Autodesk Fusion 360 part; units mm, degrees
(part 6 of 8)
  spline S293 degree 5 poles (-65.7422, 42.7079) (-65.7471, 42.7094) (-65.7716, 42.7166) (-65.8155, 42.7296) (-65.8791, 42.7481) (-65.9624, 42.7721) (-66.0605, 42.7999) (-66.1588, 42.8273) (-66.2573, 42.8543) (-66.356, 42.8809) (-66.4549, 42.9071) (-66.5539, 42.9329) (-66.6532, 42.9583) (-66.7526, 42.9833) (-66.8522, 43.008) (-66.9519, 43.0322) (-67.0519, 43.0561) (-67.152, 43.0797) (-67.2522, 43.1028) (-67.3527, 43.1256) (-67.4532, 43.148) (-67.554, 43.1701) (-67.6549, 43.1918) (-67.756, 43.2132) (-67.8572, 43.2342) (-67.9585, 43.2548) (-68.06, 43.2752) (-68.1617, 43.2951) (-68.2635, 43.3147) (-68.3654, 43.334) (-68.4675, 43.353) (-68.5697, 43.3716) (-68.6721, 43.3898) (-68.7746, 43.4078) (-68.8772, 43.4254) (-68.98, 43.4426) (-69.0829, 43.4596) (-69.1859, 43.4762) (-69.289, 43.4925) (-69.3716, 43.5053) (-69.4337, 43.5147) (-69.475, 43.521) (-69.4957, 43.524) knots 0.467834 0.467834 0.467834 0.467834 0.467834 0.467834 0.471429 0.485714 0.5 0.514286 0.528571 0.542857 0.557143 0.571429 0.585714 0.6 0.614286 0.628571 0.642857 0.657143 0.671429 0.685714 0.7 0.714286 0.728571 0.742857 0.757143 0.771429 0.785714 0.8 0.814286 0.828571 0.842857 0.857143 0.871429 0.885714 0.9 0.914286 0.928571 0.942857 0.957143 0.971429 0.985714 1 1 1 1 1 1
  arc A147 (-69.4957, 43.524) -> (-70.3306, 42.1616) centre (0, 0) ccw
  spline S294 degree 5 poles (-70.3306, 42.1616) (-70.3185, 42.1446) (-70.2941, 42.1106) (-70.2576, 42.0596) (-70.2087, 41.9918) (-70.1473, 41.9073) (-70.0857, 41.823) (-70.0239, 41.7391) (-69.9619, 41.6553) (-69.8996, 41.5719) (-69.8371, 41.4887) (-69.7743, 41.4058) (-69.7114, 41.3232) (-69.6481, 41.2408) (-69.5847, 41.1587) (-69.521, 41.0769) (-69.457, 40.9954) (-69.3929, 40.9142) (-69.3285, 40.8333) (-69.2638, 40.7526) (-69.1989, 40.6723) (-69.1337, 40.5922) (-69.0683, 40.5125) (-69.0027, 40.433) (-68.9368, 40.3539) (-68.8706, 40.2751) (-68.8042, 40.1966) (-68.7376, 40.1184) (-68.6706, 40.0405) (-68.6035, 39.963) (-68.536, 39.8857) (-68.4683, 39.8088) (-68.4004, 39.7323) (-68.3321, 39.6561) (-68.2636, 39.5802) (-68.1949, 39.5047) (-68.1258, 39.4296) (-68.0565, 39.3548) (-67.9974, 39.2915) (-67.9519, 39.2433) (-67.9204, 39.21) (-67.9029, 39.1915) (-67.8994, 39.1878) knots -1 -1 -1 -1 -1 -1 -0.985714 -0.971429 -0.957143 -0.942857 -0.928571 -0.914286 -0.9 -0.885714 -0.871429 -0.857143 -0.842857 -0.828571 -0.814286 -0.8 -0.785714 -0.771429 -0.757143 -0.742857 -0.728571 -0.714286 -0.7 -0.685714 -0.671429 -0.657143 -0.642857 -0.628571 -0.614286 -0.6 -0.585714 -0.571429 -0.557143 -0.542857 -0.528571 -0.514286 -0.5 -0.485714 -0.471429 -0.467834 -0.467834 -0.467834 -0.467834 -0.467834 -0.467834
  spline S295 degree 3 poles (-67.7523, 38.0098) (-67.6886, 38.1234) (-67.6476, 38.2483) (-67.616, 38.5068) (-67.6256, 38.6379) (-67.6817, 38.8427) (-67.7131, 38.9189) (-67.7938, 39.0619) (-67.8428, 39.1282) (-67.8994, 39.1878) knots 0 0 0 0 0.039064 0.039064 0.078129 0.078129 0.102767 0.102767 0.127404 0.127404 0.127404 0.127404
  arc A148 (-67.7523, 38.0098) -> (-67.8091, 37.9083) centre (0, 0) ccw
  spline S296 degree 3 poles (-68.8904, 37.4182) (-68.763, 37.391) (-68.6316, 37.389) (-68.3754, 37.4355) (-68.253, 37.4836) (-68.0741, 37.598) (-68.0106, 37.6506) (-67.898, 37.7701) (-67.8492, 37.8366) (-67.8091, 37.9083) knots 0 0 0 0 0.039064 0.039064 0.078129 0.078129 0.102767 0.102767 0.127404 0.127404 0.127404 0.127404
  spline S297 degree 5 poles (-68.8904, 37.4182) (-68.8954, 37.4192) (-68.9203, 37.4245) (-68.9652, 37.434) (-69.03, 37.4475) (-69.1149, 37.4649) (-69.2149, 37.4849) (-69.315, 37.5045) (-69.4153, 37.5237) (-69.5158, 37.5425) (-69.6164, 37.5608) (-69.7172, 37.5788) (-69.8182, 37.5963) (-69.9192, 37.6135) (-70.0204, 37.6302) (-70.1218, 37.6466) (-70.2233, 37.6626) (-70.3249, 37.6782) (-70.4267, 37.6934) (-70.5286, 37.7082) (-70.6307, 37.7227) (-70.7328, 37.7368) (-70.8351, 37.7505) (-70.9376, 37.7639) (-71.0401, 37.7769) (-71.1428, 37.7895) (-71.2456, 37.8018) (-71.3485, 37.8137) (-71.4515, 37.8253) (-71.5546, 37.8365) (-71.6579, 37.8474) (-71.7612, 37.8579) (-71.8647, 37.8681) (-71.9683, 37.878) (-72.072, 37.8875) (-72.1758, 37.8966) (-72.2797, 37.9054) (-72.3837, 37.9139) (-72.4878, 37.9221) (-72.5712, 37.9283) (-72.6338, 37.9329) (-72.6755, 37.9358) (-72.6964, 37.9373) knots 0.467834 0.467834 0.467834 0.467834 0.467834 0.467834 0.471429 0.485714 0.5 0.514286 0.528571 0.542857 0.557143 0.571429 0.585714 0.6 0.614286 0.628571 0.642857 0.657143 0.671429 0.685714 0.7 0.714286 0.728571 0.742857 0.757143 0.771429 0.785714 0.8 0.814286 0.828571 0.842857 0.857143 0.871429 0.885714 0.9 0.914286 0.928571 0.942857 0.957143 0.971429 0.985714 1 1 1 1 1 1
  arc A149 (-72.6964, 37.9373) -> (-73.4218, 36.5136) centre (0, 0) ccw
  spline S298 degree 5 poles (-73.4218, 36.5136) (-73.4083, 36.4976) (-73.3814, 36.4656) (-73.3409, 36.4176) (-73.2869, 36.3538) (-73.2191, 36.2744) (-73.1511, 36.1952) (-73.0829, 36.1164) (-73.0144, 36.0378) (-72.9458, 35.9595) (-72.877, 35.8815) (-72.8079, 35.8037) (-72.7386, 35.7263) (-72.6692, 35.6491) (-72.5995, 35.5723) (-72.5295, 35.4958) (-72.4594, 35.4195) (-72.389, 35.3436) (-72.3185, 35.2679) (-72.2477, 35.1926) (-72.1767, 35.1176) (-72.1054, 35.0429) (-72.034, 34.9686) (-71.9623, 34.8945) (-71.8904, 34.8208) (-71.8183, 34.7474) (-71.7459, 34.6743) (-71.6733, 34.6016) (-71.6005, 34.5292) (-71.5274, 34.4572) (-71.4541, 34.3855) (-71.3806, 34.3142) (-71.3069, 34.2432) (-71.2329, 34.1726) (-71.1586, 34.1023) (-71.0842, 34.0324) (-71.0094, 33.9629) (-70.9345, 33.8938) (-70.8705, 33.8353) (-70.8215, 33.7908) (-70.7874, 33.7601) (-70.7685, 33.7431) (-70.7647, 33.7396) knots -1 -1 -1 -1 -1 -1 -0.985714 -0.971429 -0.957143 -0.942857 -0.928571 -0.914286 -0.9 -0.885714 -0.871429 -0.857143 -0.842857 -0.828571 -0.814286 -0.8 -0.785714 -0.771429 -0.757143 -0.742857 -0.728571 -0.714286 -0.7 -0.685714 -0.671429 -0.657143 -0.642857 -0.628571 -0.614286 -0.6 -0.585714 -0.571429 -0.557143 -0.542857 -0.528571 -0.514286 -0.5 -0.485714 -0.471429 -0.467834 -0.467834 -0.467834 -0.467834 -0.467834 -0.467834
  spline S299 degree 3 poles (-70.5256, 32.5768) (-70.471, 32.695) (-70.44, 32.8228) (-70.4288, 33.083) (-70.4486, 33.2129) (-70.5206, 33.4127) (-70.5579, 33.4862) (-70.6496, 33.6225) (-70.7036, 33.6847) (-70.7647, 33.7396) knots 0 0 0 0 0.039064 0.039064 0.078129 0.078129 0.102767 0.102767 0.127404 0.127404 0.127404 0.127404
  arc A150 (-70.5256, 32.5768) -> (-70.5744, 32.4711) centre (0, 0) ccw
  spline S300 degree 3 poles (-71.6138, 31.8977) (-71.4847, 31.8807) (-71.3535, 31.889) (-71.1017, 31.9555) (-70.9835, 32.013) (-70.8142, 32.141) (-70.755, 32.1984) (-70.6521, 32.3264) (-70.6087, 32.3965) (-70.5744, 32.4711) knots 0 0 0 0 0.039064 0.039064 0.078129 0.078129 0.102767 0.102767 0.127404 0.127404 0.127404 0.127404
  spline S301 degree 5 poles (-71.6138, 31.8977) (-71.6189, 31.8984) (-71.6442, 31.9018) (-71.6896, 31.9077) (-71.7553, 31.9161) (-71.8413, 31.9267) (-71.9425, 31.9389) (-72.0439, 31.9505) (-72.1454, 31.9618) (-72.2471, 31.9726) (-72.3488, 31.983) (-72.4507, 31.993) (-72.5527, 32.0026) (-72.6548, 32.0117) (-72.757, 32.0205) (-72.8594, 32.0289) (-72.9618, 32.0368) (-73.0644, 32.0444) (-73.167, 32.0516) (-73.2698, 32.0584) (-73.3726, 32.0648) (-73.4756, 32.0708) (-73.5786, 32.0765) (-73.6818, 32.0818) (-73.785, 32.0867) (-73.8884, 32.0912) (-73.9918, 32.0954) (-74.0953, 32.0992) (-74.199, 32.1027) (-74.3027, 32.1058) (-74.4065, 32.1085) (-74.5103, 32.1109) (-74.6143, 32.1129) (-74.7183, 32.1146) (-74.8224, 32.116) (-74.9266, 32.1169) (-75.0309, 32.1176) (-75.1353, 32.1179) (-75.2397, 32.1178) (-75.3233, 32.1175) (-75.386, 32.1172) (-75.4279, 32.1168) (-75.4488, 32.1167) knots 0.467834 0.467834 0.467834 0.467834 0.467834 0.467834 0.471429 0.485714 0.5 0.514286 0.528571 0.542857 0.557143 0.571429 0.585714 0.6 0.614286 0.628571 0.642857 0.657143 0.671429 0.685714 0.7 0.714286 0.728571 0.742857 0.757143 0.771429 0.785714 0.8 0.814286 0.828571 0.842857 0.857143 0.871429 0.885714 0.9 0.914286 0.928571 0.942857 0.957143 0.971429 0.985714 1 1 1 1 1 1
  arc A151 (-75.4488, 32.1167) -> (-76.0603, 30.6404) centre (0, 0) ccw
  spline S302 degree 5 poles (-76.0603, 30.6404) (-76.0456, 30.6255) (-76.0162, 30.5957) (-75.9721, 30.5511) (-75.9132, 30.4917) (-75.8394, 30.4179) (-75.7654, 30.3443) (-75.6912, 30.271) (-75.6169, 30.198) (-75.5423, 30.1254) (-75.4675, 30.053) (-75.3926, 29.9809) (-75.3175, 29.9091) (-75.2421, 29.8377) (-75.1666, 29.7666) (-75.0909, 29.6957) (-75.015, 29.6252) (-74.9389, 29.555) (-74.8626, 29.4852) (-74.7861, 29.4156) (-74.7095, 29.3464) (-74.6326, 29.2776) (-74.5555, 29.209) (-74.4783, 29.1408) (-74.4008, 29.073) (-74.3231, 29.0055) (-74.2452, 28.9383) (-74.1672, 28.8715) (-74.0889, 28.8051) (-74.0104, 28.739) (-73.9317, 28.6733) (-73.8528, 28.6079) (-73.7737, 28.543) (-73.6944, 28.4784) (-73.6149, 28.4141) (-73.5352, 28.3503) (-73.4552, 28.2869) (-73.3751, 28.2238) (-73.3067, 28.1706) (-73.2543, 28.1301) (-73.218, 28.1021) (-73.1978, 28.0866) (-73.1937, 28.0835) knots -1 -1 -1 -1 -1 -1 -0.985714 -0.971429 -0.957143 -0.942857 -0.928571 -0.914286 -0.9 -0.885714 -0.871429 -0.857143 -0.842857 -0.828571 -0.814286 -0.8 -0.785714 -0.771429 -0.757143 -0.742857 -0.728571 -0.714286 -0.7 -0.685714 -0.671429 -0.657143 -0.642857 -0.628571 -0.614286 -0.6 -0.585714 -0.571429 -0.557143 -0.542857 -0.528571 -0.514286 -0.5 -0.485714 -0.471429 -0.467834 -0.467834 -0.467834 -0.467834 -0.467834 -0.467834
  spline S303 degree 3 poles (-72.8642, 26.943) (-72.819, 27.0652) (-72.7981, 27.195) (-72.8073, 27.4552) (-72.8373, 27.5832) (-72.9248, 27.7767) (-72.9677, 27.8471) (-73.0698, 27.9757) (-73.1286, 28.0335) (-73.1937, 28.0835) knots 0 0 0 0 0.039064 0.039064 0.078129 0.078129 0.102767 0.102767 0.127404 0.127404 0.127404 0.127404
  arc A152 (-72.8642, 26.943) -> (-72.9045, 26.8339) centre (0, 0) ccw
  spline S304 degree 3 poles (-73.8957, 26.1807) (-73.7657, 26.1738) (-73.6356, 26.1924) (-73.3897, 26.2784) (-73.2764, 26.345) (-73.1176, 26.4859) (-73.0631, 26.5478) (-72.9706, 26.6835) (-72.9328, 26.7568) (-72.9045, 26.8339) knots 0 0 0 0 0.039064 0.039064 0.078129 0.078129 0.102767 0.102767 0.127404 0.127404 0.127404 0.127404
  spline S305 degree 5 poles (-73.8957, 26.1807) (-73.9008, 26.1809) (-73.9263, 26.1823) (-73.9721, 26.1846) (-74.0382, 26.1878) (-74.1248, 26.1917) (-74.2267, 26.1959) (-74.3286, 26.1995) (-74.4307, 26.2028) (-74.5329, 26.2056) (-74.6352, 26.208) (-74.7375, 26.2099) (-74.8399, 26.2115) (-74.9424, 26.2126) (-75.045, 26.2133) (-75.1477, 26.2136) (-75.2505, 26.2136) (-75.3533, 26.2131) (-75.4562, 26.2122) (-75.5592, 26.2109) (-75.6622, 26.2092) (-75.7653, 26.2072) (-75.8685, 26.2047) (-75.9718, 26.2019) (-76.0751, 26.1987) (-76.1785, 26.1951) (-76.2819, 26.1912) (-76.3854, 26.1868) (-76.489, 26.1821) (-76.5926, 26.1771) (-76.6963, 26.1717) (-76.8, 26.1659) (-76.9038, 26.1598) (-77.0077, 26.1533) (-77.1116, 26.1464) (-77.2155, 26.1393) (-77.3195, 26.1317) (-77.4236, 26.1238) (-77.5277, 26.1156) (-77.611, 26.1087) (-77.6735, 26.1034) (-77.7152, 26.0998) (-77.736, 26.098) knots 0.467834 0.467834 0.467834 0.467834 0.467834 0.467834 0.471429 0.485714 0.5 0.514286 0.528571 0.542857 0.557143 0.571429 0.585714 0.6 0.614286 0.628571 0.642857 0.657143 0.671429 0.685714 0.7 0.714286 0.728571 0.742857 0.757143 0.771429 0.785714 0.8 0.814286 0.828571 0.842857 0.857143 0.871429 0.885714 0.9 0.914286 0.928571 0.942857 0.957143 0.971429 0.985714 1 1 1 1 1 1
  arc A153 (-77.736, 26.098) -> (-78.2298, 24.5784) centre (0, 0) ccw
  spline S306 degree 5 poles (-78.2298, 24.5784) (-78.214, 24.5646) (-78.1824, 24.5372) (-78.135, 24.4962) (-78.0716, 24.4417) (-77.9922, 24.3738) (-77.9127, 24.3063) (-77.8329, 24.239) (-77.7531, 24.1721) (-77.673, 24.1055) (-77.5928, 24.0392) (-77.5125, 23.9733) (-77.4319, 23.9076) (-77.3512, 23.8423) (-77.2704, 23.7773) (-77.1893, 23.7126) (-77.1081, 23.6483) (-77.0268, 23.5843) (-76.9452, 23.5206) (-76.8635, 23.4573) (-76.7817, 23.3943) (-76.6996, 23.3317) (-76.6174, 23.2694) (-76.535, 23.2075) (-76.4525, 23.1459) (-76.3697, 23.0847) (-76.2868, 23.0239) (-76.2038, 22.9634) (-76.1205, 22.9033) (-76.0371, 22.8436) (-75.9535, 22.7843) (-75.8697, 22.7253) (-75.7858, 22.6667) (-75.7016, 22.6086) (-75.6173, 22.5508) (-75.5328, 22.4934) (-75.4482, 22.4364) (-75.3633, 22.3799) (-75.291, 22.3322) (-75.2356, 22.2959) (-75.1972, 22.2709) (-75.1758, 22.257) (-75.1715, 22.2542) knots -1 -1 -1 -1 -1 -1 -0.985714 -0.971429 -0.957143 -0.942857 -0.928571 -0.914286 -0.9 -0.885714 -0.871429 -0.857143 -0.842857 -0.828571 -0.814286 -0.8 -0.785714 -0.771429 -0.757143 -0.742857 -0.728571 -0.714286 -0.7 -0.685714 -0.671429 -0.657143 -0.642857 -0.628571 -0.614286 -0.6 -0.585714 -0.571429 -0.557143 -0.542857 -0.528571 -0.514286 -0.5 -0.485714 -0.471429 -0.467834 -0.467834 -0.467834 -0.467834 -0.467834 -0.467834
  spline S307 degree 3 poles (-74.7535, 21.1431) (-74.718, 21.2684) (-74.7074, 21.3994) (-74.737, 21.6582) (-74.7769, 21.7834) (-74.8793, 21.9695) (-74.9276, 22.0363) (-75.0395, 22.1565) (-75.1026, 22.2095) (-75.1715, 22.2542) knots 0 0 0 0 0.039064 0.039064 0.078129 0.078129 0.102767 0.102767 0.127404 0.127404 0.127404 0.127404
  arc A154 (-74.7535, 21.1431) -> (-74.7851, 21.0311) centre (0, 0) ccw
  spline S308 degree 3 poles (-75.722, 20.3022) (-75.5919, 20.3055) (-75.4636, 20.3342) (-75.2253, 20.4393) (-75.1175, 20.5146) (-74.9703, 20.6675) (-74.9208, 20.7335) (-74.8392, 20.876) (-74.8073, 20.9521) (-74.7851, 21.0311) knots 0 0 0 0 0.039064 0.039064 0.078129 0.078129 0.102767 0.102767 0.127404 0.127404 0.127404 0.127404
  spline S309 degree 5 poles (-75.722, 20.3022) (-75.7272, 20.302) (-75.7526, 20.3014) (-75.7985, 20.3001) (-75.8646, 20.2981) (-75.9512, 20.2952) (-76.0531, 20.2913) (-76.1551, 20.287) (-76.2571, 20.2822) (-76.3592, 20.277) (-76.4613, 20.2714) (-76.5635, 20.2653) (-76.6658, 20.2588) (-76.768, 20.2519) (-76.8704, 20.2446) (-76.9728, 20.2368) (-77.0752, 20.2287) (-77.1777, 20.2201) (-77.2802, 20.2111) (-77.3827, 20.2018) (-77.4853, 20.192) (-77.588, 20.1819) (-77.6906, 20.1714) (-77.7934, 20.1604) (-77.8961, 20.1491) (-77.9989, 20.1375) (-78.1017, 20.1254) (-78.2045, 20.113) (-78.3074, 20.1002) (-78.4103, 20.087) (-78.5133, 20.0735) (-78.6162, 20.0596) (-78.7192, 20.0453) (-78.8222, 20.0307) (-78.9253, 20.0157) (-79.0284, 20.0004) (-79.1314, 19.9847) (-79.2346, 19.9687) (-79.3377, 19.9523) (-79.4202, 19.939) (-79.4821, 19.9288) (-79.5234, 19.9219) (-79.544, 19.9185) knots 0.467834 0.467834 0.467834 0.467834 0.467834 0.467834 0.471429 0.485714 0.5 0.514286 0.528571 0.542857 0.557143 0.571429 0.585714 0.6 0.614286 0.628571 0.642857 0.657143 0.671429 0.685714 0.7 0.714286 0.728571 0.742857 0.757143 0.771429 0.785714 0.8 0.814286 0.828571 0.842857 0.857143 0.871429 0.885714 0.9 0.914286 0.928571 0.942857 0.957143 0.971429 0.985714 1 1 1 1 1 1
  arc A155 (-79.544, 19.9185) -> (-79.9171, 18.3648) centre (0, 0) ccw
  spline S310 degree 5 poles (-79.9171, 18.3648) (-79.9002, 18.3523) (-79.8666, 18.3275) (-79.816, 18.2903) (-79.7486, 18.2409) (-79.6641, 18.1795) (-79.5795, 18.1184) (-79.4948, 18.0576) (-79.4099, 17.9972) (-79.3249, 17.9371) (-79.2397, 17.8773) (-79.1544, 17.8178) (-79.069, 17.7587) (-78.9834, 17.6999) (-78.8977, 17.6414) (-78.8119, 17.5833) (-78.7259, 17.5256) (-78.6397, 17.4681) (-78.5534, 17.4111) (-78.467, 17.3544) (-78.3805, 17.298) (-78.2938, 17.242) (-78.2069, 17.1864) (-78.1199, 17.1311) (-78.0328, 17.0762) (-77.9455, 17.0217) (-77.8581, 16.9675) (-77.7706, 16.9138) (-77.6828, 16.8604) (-77.595, 16.8074) (-77.507, 16.7548) (-77.4189, 16.7026) (-77.3306, 16.6508) (-77.2421, 16.5994) (-77.1535, 16.5484) (-77.0648, 16.4978) (-76.9759, 16.4477) (-76.8869, 16.398) (-76.8111, 16.3561) (-76.753, 16.3242) (-76.7127, 16.3023) (-76.6903, 16.2902) (-76.6858, 16.2877) knots -1 -1 -1 -1 -1 -1 -0.985714 -0.971429 -0.957143 -0.942857 -0.928571 -0.914286 -0.9 -0.885714 -0.871429 -0.857143 -0.842857 -0.828571 -0.814286 -0.8 -0.785714 -0.771429 -0.757143 -0.742857 -0.728571 -0.714286 -0.7 -0.685714 -0.671429 -0.657143 -0.642857 -0.628571 -0.614286 -0.6 -0.585714 -0.571429 -0.557143 -0.542857 -0.528571 -0.514286 -0.5 -0.485714 -0.471429 -0.467834 -0.467834 -0.467834 -0.467834 -0.467834 -0.467834
  spline S311 degree 3 poles (-76.1819, 15.2129) (-76.1564, 15.3405) (-76.1561, 15.472) (-76.2059, 15.7276) (-76.2555, 15.8494) (-76.3722, 16.0268) (-76.4256, 16.0896) (-76.5465, 16.2007) (-76.6136, 16.2486) (-76.6858, 16.2877) knots 0 0 0 0 0.039064 0.039064 0.078129 0.078129 0.102767 0.102767 0.127404 0.127404 0.127404 0.127404
  arc A156 (-76.1819, 15.2129) -> (-76.2046, 15.0987) centre (0, 0) ccw
  spline S312 degree 3 poles (-77.0815, 14.2985) (-76.952, 14.312) (-76.8264, 14.3508) (-76.597, 14.4742) (-76.4955, 14.5577) (-76.3607, 14.7217) (-76.3166, 14.7914) (-76.2464, 14.9399) (-76.2206, 15.0182) (-76.2046, 15.0987) knots 0 0 0 0 0.039064 0.039064 0.078129 0.078129 0.102767 0.102767 0.127404 0.127404 0.127404 0.127404
  spline S313 degree 5 poles (-77.0815, 14.2985) (-77.0866, 14.298) (-77.1119, 14.2953) (-77.1575, 14.2905) (-77.2234, 14.2833) (-77.3095, 14.2736) (-77.4107, 14.2617) (-77.512, 14.2494) (-77.6134, 14.2367) (-77.7147, 14.2234) (-77.8161, 14.2098) (-77.9175, 14.1957) (-78.0189, 14.1812) (-78.1203, 14.1663) (-78.2218, 14.151) (-78.3232, 14.1352) (-78.4247, 14.1191) (-78.5262, 14.1025) (-78.6277, 14.0855) (-78.7292, 14.0681) (-78.8307, 14.0504) (-78.9322, 14.0322) (-79.0338, 14.0136) (-79.1353, 13.9947) (-79.2369, 13.9754) (-79.3384, 13.9557) (-79.44, 13.9356) (-79.5415, 13.9151) (-79.6431, 13.8943) (-79.7446, 13.8731) (-79.8462, 13.8515) (-79.9477, 13.8296) (-80.0493, 13.8073) (-80.1509, 13.7846) (-80.2524, 13.7616) (-80.354, 13.7383) (-80.4555, 13.7146) (-80.557, 13.6905) (-80.6586, 13.6661) (-80.7398, 13.6463) (-80.8007, 13.6312) (-80.8413, 13.6212) (-80.8616, 13.6161) knots 0.467834 0.467834 0.467834 0.467834 0.467834 0.467834 0.471429 0.485714 0.5 0.514286 0.528571 0.542857 0.557143 0.571429 0.585714 0.6 0.614286 0.628571 0.642857 0.657143 0.671429 0.685714 0.7 0.714286 0.728571 0.742857 0.757143 0.771429 0.785714 0.8 0.814286 0.828571 0.842857 0.857143 0.871429 0.885714 0.9 0.914286 0.928571 0.942857 0.957143 0.971429 0.985714 1 1 1 1 1 1
  arc A157 (-80.8616, 13.6161) -> (-81.1116, 12.0379) centre (0, 0) ccw
  spline S314 degree 5 poles (-81.1116, 12.0379) (-81.0938, 12.0268) (-81.0583, 12.0047) (-81.005, 11.9716) (-80.9339, 11.9277) (-80.8449, 11.8731) (-80.7558, 11.8188) (-80.6665, 11.7649) (-80.5772, 11.7113) (-80.4877, 11.658) (-80.3981, 11.6051) (-80.3084, 11.5525) (-80.2186, 11.5002) (-80.1287, 11.4483) (-80.0386, 11.3968) (-79.9485, 11.3456) (-79.8582, 11.2948) (-79.7678, 11.2443) (-79.6774, 11.1942) (-79.5867, 11.1444) (-79.496, 11.095) (-79.4052, 11.046) (-79.3143, 10.9973) (-79.2232, 10.9491) (-79.132, 10.9012) (-79.0408, 10.8537) (-78.9494, 10.8066) (-78.8579, 10.7598) (-78.7662, 10.7135) (-78.6745, 10.6675) (-78.5826, 10.622) (-78.4907, 10.5769) (-78.3986, 10.5322) (-78.3064, 10.4879) (-78.2141, 10.444) (-78.1217, 10.4005) (-78.0291, 10.3575) (-77.9364, 10.3149) (-77.8576, 10.2791) (-77.7972, 10.252) (-77.7553, 10.2333) (-77.732, 10.2229) (-77.7274, 10.2208) knots -1 -1 -1 -1 -1 -1 -0.985714 -0.971429 -0.957143 -0.942857 -0.928571 -0.914286 -0.9 -0.885714 -0.871429 -0.857143 -0.842857 -0.828571 -0.814286 -0.8 -0.785714 -0.771429 -0.757143 -0.742857 -0.728571 -0.714286 -0.7 -0.685714 -0.671429 -0.657143 -0.642857 -0.628571 -0.614286 -0.6 -0.585714 -0.571429 -0.557143 -0.542857 -0.528571 -0.514286 -0.5 -0.485714 -0.471429 -0.467834 -0.467834 -0.467834 -0.467834 -0.467834 -0.467834
  spline S315 degree 3 poles (-77.1407, 9.1888) (-77.1253, 9.3181) (-77.1353, 9.4492) (-77.2049, 9.7001) (-77.2639, 9.8176) (-77.3942, 9.9853) (-77.4524, 10.0437) (-77.5817, 10.145) (-77.6523, 10.1875) (-77.7274, 10.2208) knots 0 0 0 0 0.039064 0.039064 0.078129 0.078129 0.102767 0.102767 0.127404 0.127404 0.127404 0.127404
  arc A158 (-77.1407, 9.1888) -> (-77.1543, 9.0732) centre (0, 0) ccw
  spline S316 degree 3 poles (-77.9657, 8.2067) (-77.8377, 8.2303) (-77.7155, 8.2788) (-77.4965, 8.4198) (-77.4019, 8.511) (-77.2804, 8.6852) (-77.2419, 8.758) (-77.1835, 8.9116) (-77.1639, 8.9917) (-77.1543, 9.0732) knots 0 0 0 0 0.039064 0.039064 0.078129 0.078129 0.102767 0.102767 0.127404 0.127404 0.127404 0.127404
  spline S317 degree 5 poles (-77.9657, 8.2067) (-77.9708, 8.2057) (-77.9958, 8.2011) (-78.0409, 8.1927) (-78.106, 8.1804) (-78.191, 8.164) (-78.2911, 8.1442) (-78.3911, 8.124) (-78.4911, 8.1033) (-78.5911, 8.0822) (-78.6911, 8.0606) (-78.7911, 8.0386) (-78.8911, 8.0162) (-78.991, 7.9934) (-79.0909, 7.9701) (-79.1908, 7.9465) (-79.2907, 7.9224) (-79.3906, 7.8979) (-79.4904, 7.873) (-79.5903, 7.8477) (-79.6901, 7.8221) (-79.7899, 7.796) (-79.8896, 7.7695) (-79.9894, 7.7427) (-80.0891, 7.7154) (-80.1888, 7.6878) (-80.2884, 7.6598) (-80.3881, 7.6315) (-80.4877, 7.6027) (-80.5873, 7.5736) (-80.6868, 7.5442) (-80.7863, 7.5143) (-80.8858, 7.4841) (-80.9853, 7.4536) (-81.0847, 7.4227) (-81.1841, 7.3914) (-81.2835, 7.3598) (-81.3828, 7.3279) (-81.4822, 7.2955) (-81.5616, 7.2694) (-81.6211, 7.2497) (-81.6608, 7.2364) (-81.6807, 7.2298) knots 0.467834 0.467834 0.467834 0.467834 0.467834 0.467834 0.471429 0.485714 0.5 0.514286 0.528571 0.542857 0.557143 0.571429 0.585714 0.6 0.614286 0.628571 0.642857 0.657143 0.671429 0.685714 0.7 0.714286 0.728571 0.742857 0.757143 0.771429 0.785714 0.8 0.814286 0.828571 0.842857 0.857143 0.871429 0.885714 0.9 0.914286 0.928571 0.942857 0.957143 0.971429 0.985714 1 1 1 1 1 1
  arc A159 (-81.6807, 7.2298) -> (-81.806, 5.6369) centre (0, 0) ccw
  spline S318 degree 5 poles (-81.806, 5.6369) (-81.7875, 5.6272) (-81.7503, 5.6079) (-81.6946, 5.5791) (-81.6202, 5.5409) (-81.5272, 5.4934) (-81.4341, 5.4463) (-81.3409, 5.3996) (-81.2476, 5.3532) (-81.1542, 5.3071) (-81.0608, 5.2613) (-80.9672, 5.216) (-80.8736, 5.1709) (-80.7799, 5.1262) (-80.6861, 5.0819) (-80.5922, 5.038) (-80.4982, 4.9943) (-80.4042, 4.9511) (-80.31, 4.9082) (-80.2158, 4.8658) (-80.1215, 4.8236) (-80.0271, 4.7819) (-79.9326, 4.7405) (-79.838, 4.6995) (-79.7434, 4.6589) (-79.6487, 4.6187) (-79.5539, 4.5789) (-79.459, 4.5395) (-79.364, 4.5005) (-79.2689, 4.4619) (-79.1738, 4.4237) (-79.0786, 4.386) (-78.9833, 4.3486) (-78.8879, 4.3117) (-78.7924, 4.2752) (-78.6968, 4.2391) (-78.6012, 4.2035) (-78.5055, 4.1683) (-78.424, 4.1388) (-78.3617, 4.1165) (-78.3185, 4.1011) (-78.2945, 4.0926) (-78.2897, 4.0909) knots -1 -1 -1 -1 -1 -1 -0.985714 -0.971429 -0.957143 -0.942857 -0.928571 -0.914286 -0.9 -0.885714 -0.871429 -0.857143 -0.842857 -0.828571 -0.814286 -0.8 -0.785714 -0.771429 -0.757143 -0.742857 -0.728571 -0.714286 -0.7 -0.685714 -0.671429 -0.657143 -0.642857 -0.628571 -0.614286 -0.6 -0.585714 -0.571429 -0.557143 -0.542857 -0.528571 -0.514286 -0.5 -0.485714 -0.471429 -0.467834 -0.467834 -0.467834 -0.467834 -0.467834 -0.467834
  spline S319 degree 3 poles (-77.6238, 3.1081) (-77.6186, 3.2382) (-77.6388, 3.3681) (-77.728, 3.6128) (-77.796, 3.7252) (-77.939, 3.8822) (-78.0016, 3.9359) (-78.1385, 4.0267) (-78.2122, 4.0635) (-78.2897, 4.0909) knots 0 0 0 0 0.039064 0.039064 0.078129 0.078129 0.102767 0.102767 0.127404 0.127404 0.127404 0.127404
  circle A160 centre (0, 0) radius 90
  dimension "d9" = 180
  constraint coincident A0.centre A1.centre
  measures "d9" diameter of A160
extrude "Extrude1" add sketch "Sketch1" against normal blind 10 makes body 1 in component "Ring gear"
sketch "Base Circle" plane through (0, 0, 0) normal (0, 0, 1) x (1, 0, 0) in component "Planetary Gear"
  circle A0 centre (0, 0) radius 29.686
  circle A1 centre (0, 0) radius 2.5
extrude "Extrude1'" add sketch "Base Circle" along normal blind 10 separate body makes body 2 in component "Planetary Gear"
sketch "Gear Tooth" plane through (0, 0, 0) normal (0, 0, 1) x (1, 0, 0) in component "Planetary Gear"
  spline S0 degree 5 poles (30.0159, -1.8057) (30.0274, -1.8064) (30.0503, -1.8075) (30.0848, -1.8084) (30.1307, -1.808) (30.1881, -1.8055) (30.2456, -1.8015) (30.3031, -1.7965) (30.3606, -1.7911) (30.4181, -1.7853) (30.4756, -1.7791) (30.5331, -1.7725) (30.5906, -1.7653) (30.6481, -1.7574) (30.7056, -1.7488) (30.7631, -1.7395) (30.8206, -1.7296) (30.878, -1.7192) (30.9355, -1.7084) (30.9929, -1.6972) (31.0503, -1.6856) (31.1077, -1.6736) (31.1651, -1.6612) (31.2225, -1.6483) (31.2798, -1.635) (31.3371, -1.6213) (31.3944, -1.6072) (31.4517, -1.5926) (31.509, -1.5777) (31.5662, -1.5625) (31.6234, -1.5469) (31.6806, -1.5309) (31.7377, -1.5146) (31.7949, -1.4979) (31.852, -1.4809) (31.909, -1.4635) (31.9661, -1.4458) (32.0231, -1.4278) (32.08, -1.4094) (32.137, -1.3907) (32.1939, -1.3717) (32.2508, -1.3523) (32.3076, -1.3327) (32.3644, -1.3127) (32.4212, -1.2925) (32.478, -1.2719) (32.5347, -1.251) (32.5913, -1.2299) (32.648, -1.2084) (32.7046, -1.1866) (32.7611, -1.1646) (32.8176, -1.1423) (32.8741, -1.1196) (32.9305, -1.0967) (32.9869, -1.0735) (33.0433, -1.0501) (33.0996, -1.0263) (33.1559, -1.0023) (33.2121, -0.978) (33.2683, -0.9535) (33.3244, -0.9286) (33.3805, -0.9035) (33.4366, -0.8782) (33.4926, -0.8525) (33.5486, -0.8266) (33.6045, -0.8005) (33.6603, -0.7741) (33.7162, -0.7474) (33.7719, -0.7205) (33.8277, -0.6933) (33.8833, -0.6659) (33.9278, -0.6438) (33.9612, -0.627) (33.9834, -0.6158) (33.9945, -0.6102) knots 0 0 0 0 0 0 0.01428571 0.02857143 0.04285714 0.05714286 0.07142857 0.08571429 0.1 0.11428571 0.12857143 0.14285714 0.15714286 0.17142857 0.18571429 0.2 0.21428571 0.22857143 0.24285714 0.25714286 0.27142857 0.28571429 0.3 0.31428571 0.32857143 0.34285714 0.35714286 0.37142857 0.38571429 0.4 0.41428571 0.42857143 0.44285714 0.45714286 0.47142857 0.48571429 0.5 0.51428571 0.52857143 0.54285714 0.55714286 0.57142857 0.58571429 0.6 0.61428571 0.62857143 0.64285714 0.65714286 0.67142857 0.68571429 0.7 0.71428571 0.72857143 0.74285714 0.75714286 0.77142857 0.78571429 0.8 0.81428571 0.82857143 0.84285714 0.85714286 0.87142857 0.88571429 0.9 0.91428571 0.92857143 0.94285714 0.95714286 0.97142857 0.98571429 1 1 1 1 1 1
  spline S1 degree 5 poles (30.0159, 1.8057) (30.0274, 1.8064) (30.0503, 1.8075) (30.0848, 1.8084) (30.1307, 1.808) (30.1881, 1.8055) (30.2456, 1.8015) (30.3031, 1.7965) (30.3606, 1.7911) (30.4181, 1.7853) (30.4756, 1.7791) (30.5331, 1.7725) (30.5906, 1.7653) (30.6481, 1.7574) (30.7056, 1.7488) (30.7631, 1.7395) (30.8206, 1.7296) (30.878, 1.7192) (30.9355, 1.7084) (30.9929, 1.6972) (31.0503, 1.6856) (31.1077, 1.6736) (31.1651, 1.6612) (31.2225, 1.6483) (31.2798, 1.635) (31.3371, 1.6213) (31.3944, 1.6072) (31.4517, 1.5926) (31.509, 1.5777) (31.5662, 1.5625) (31.6234, 1.5469) (31.6806, 1.5309) (31.7377, 1.5146) (31.7949, 1.4979) (31.852, 1.4809) (31.909, 1.4635) (31.9661, 1.4458) (32.0231, 1.4278) (32.08, 1.4094) (32.137, 1.3907) (32.1939, 1.3717) (32.2508, 1.3523) (32.3076, 1.3327) (32.3644, 1.3127) (32.4212, 1.2925) (32.478, 1.2719) (32.5347, 1.251) (32.5913, 1.2299) (32.648, 1.2084) (32.7046, 1.1866) (32.7611, 1.1646) (32.8176, 1.1423) (32.8741, 1.1196) (32.9305, 1.0967) (32.9869, 1.0735) (33.0433, 1.0501) (33.0996, 1.0263) (33.1559, 1.0023) (33.2121, 0.978) (33.2683, 0.9535) (33.3244, 0.9286) (33.3805, 0.9035) (33.4366, 0.8782) (33.4926, 0.8525) (33.5486, 0.8266) (33.6045, 0.8005) (33.6603, 0.7741) (33.7162, 0.7474) (33.7719, 0.7205) (33.8277, 0.6933) (33.8833, 0.6659) (33.9278, 0.6438) (33.9612, 0.627) (33.9834, 0.6158) (33.9945, 0.6102) knots 0 0 0 0 0 0 0.01428571 0.02857143 0.04285714 0.05714286 0.07142857 0.08571429 0.1 0.11428571 0.12857143 0.14285714 0.15714286 0.17142857 0.18571429 0.2 0.21428571 0.22857143 0.24285714 0.25714286 0.27142857 0.28571429 0.3 0.31428571 0.32857143 0.34285714 0.35714286 0.37142857 0.38571429 0.4 0.41428571 0.42857143 0.44285714 0.45714286 0.47142857 0.48571429 0.5 0.51428571 0.52857143 0.54285714 0.55714286 0.57142857 0.58571429 0.6 0.61428571 0.62857143 0.64285714 0.65714286 0.67142857 0.68571429 0.7 0.71428571 0.72857143 0.74285714 0.75714286 0.77142857 0.78571429 0.8 0.81428571 0.82857143 0.84285714 0.85714286 0.87142857 0.88571429 0.9 0.91428571 0.92857143 0.94285714 0.95714286 0.97142857 0.98571429 1 1 1 1 1 1
  arc A0 (33.9945, -0.6102) -> (33.9945, 0.6102) centre (0, 0) ccw
  line L0 (29.6224, -1.782) -> (30.0159, -1.8057)
  line L1 (29.6224, 1.782) -> (30.0159, 1.8057)
  line L2 (29.6224, -1.782) -> (29.6224, 1.782)
  point P0 (30.2976, -1.7969)
  point P1 (30.5806, -1.7665)
  point P2 (30.8643, -1.7216)
  point P3 (31.1485, -1.6647)
  point P4 (31.4331, -1.5973)
  point P5 (31.718, -1.5202)
  point P6 (32.003, -1.4341)
  point P7 (32.288, -1.3394)
  point P8 (32.573, -1.2367)
  point P9 (32.8579, -1.1261)
  point P10 (33.1426, -1.0079)
  point P11 (33.4269, -0.8825)
  point P12 (33.711, -0.7498)
  point P13 (30.2976, 1.7969)
  point P14 (30.5806, 1.7665)
  point P15 (30.8643, 1.7216)
  point P16 (31.1485, 1.6647)
  point P17 (31.4331, 1.5973)
  point P18 (31.718, 1.5202)
  point P19 (32.003, 1.4341)
  point P20 (32.288, 1.3394)
  point P21 (32.573, 1.2367)
  point P22 (32.8579, 1.1261)
  point P23 (33.1426, 1.0079)
  point P24 (33.4269, 0.8825)
  point P25 (33.711, 0.7498)
extrude "Extrude2" add sketch "Gear Tooth" along normal blind 10 bodies 2 in component "Planetary Gear"
fillet "Fillet1" radius 1 2 edges at (29.6324, -1.7826, 5) (29.6324, 1.7826, 5) on bodies 2 in component "Planetary Gear"
pattern_circular "C-Pattern1" count 32 over 360 about axis through (0, 0, 0) along (0, 0, 1) of "Extrude2", "Fillet1" in component "Planetary Gear"
sketch "Diametrial Pitch Circle" plane through (0, 0, 0) normal (0, 0, 1) x (1, 0, 0) in component "Planetary Gear"
  circle A0 centre (0, 0) radius 32 construction
sketch "Base Circle (2)" plane through (0, 0, 0) normal (0, 0, 1) x (1, 0, 0) in component "Sun Gear"
  circle A0 centre (0, 0) radius 13.686
  circle A1 centre (0, 0) radius 2.5
extrude "Extrude1''" add sketch "Base Circle (2)" along normal blind 10 separate body makes body 3 in component "Sun Gear"
sketch "Gear Tooth (2)" plane through (0, 0, 0) normal (0, 0, 1) x (1, 0, 0) in component "Sun Gear"
  spline S0 degree 5 poles (14.9519, -1.5798) (14.9606, -1.5807) (14.978, -1.5823) (15.0041, -1.5839) (15.039, -1.5847) (15.0828, -1.5837) (15.1266, -1.5812) (15.1705, -1.578) (15.2144, -1.5742) (15.2583, -1.5701) (15.3023, -1.5657) (15.3463, -1.5609) (15.3903, -1.5554) (15.4343, -1.5493) (15.4783, -1.5425) (15.5224, -1.535) (15.5664, -1.527) (15.6104, -1.5186) (15.6545, -1.5097) (15.6985, -1.5005) (15.7425, -1.4909) (15.7866, -1.4808) (15.8306, -1.4704) (15.8746, -1.4595) (15.9186, -1.4482) (15.9626, -1.4365) (16.0065, -1.4244) (16.0505, -1.4119) (16.0944, -1.3991) (16.1383, -1.3859) (16.1822, -1.3724) (16.2261, -1.3585) (16.2699, -1.3443) (16.3137, -1.3297) (16.3575, -1.3147) (16.4013, -1.2995) (16.4451, -1.2839) (16.4888, -1.2679) (16.5324, -1.2517) (16.5761, -1.2351) (16.6197, -1.2182) (16.6633, -1.201) (16.7068, -1.1835) (16.7504, -1.1657) (16.7938, -1.1475) (16.8373, -1.1291) (16.8807, -1.1104) (16.924, -1.0913) (16.9674, -1.072) (17.0106, -1.0524) (17.0539, -1.0325) (17.0971, -1.0123) (17.1402, -0.9918) (17.1833, -0.9711) (17.2264, -0.95) (17.2694, -0.9287) (17.3123, -0.9071) (17.3552, -0.8852) (17.3981, -0.863) (17.4409, -0.8406) (17.4837, -0.8179) (17.5264, -0.795) (17.569, -0.7717) (17.6116, -0.7482) (17.6541, -0.7245) (17.6966, -0.7004) (17.7391, -0.6762) (17.7814, -0.6516) (17.8237, -0.6268) (17.866, -0.6018) (17.9082, -0.5765) (17.9419, -0.556) (17.9671, -0.5405) (17.9839, -0.5302) (17.9923, -0.525) knots 0 0 0 0 0 0 0.01428571 0.02857143 0.04285714 0.05714286 0.07142857 0.08571429 0.1 0.11428571 0.12857143 0.14285714 0.15714286 0.17142857 0.18571429 0.2 0.21428571 0.22857143 0.24285714 0.25714286 0.27142857 0.28571429 0.3 0.31428571 0.32857143 0.34285714 0.35714286 0.37142857 0.38571429 0.4 0.41428571 0.42857143 0.44285714 0.45714286 0.47142857 0.48571429 0.5 0.51428571 0.52857143 0.54285714 0.55714286 0.57142857 0.58571429 0.6 0.61428571 0.62857143 0.64285714 0.65714286 0.67142857 0.68571429 0.7 0.71428571 0.72857143 0.74285714 0.75714286 0.77142857 0.78571429 0.8 0.81428571 0.82857143 0.84285714 0.85714286 0.87142857 0.88571429 0.9 0.91428571 0.92857143 0.94285714 0.95714286 0.97142857 0.98571429 1 1 1 1 1 1
  spline S1 degree 5 poles (14.9519, 1.5798) (14.9606, 1.5807) (14.978, 1.5823) (15.0041, 1.5839) (15.039, 1.5847) (15.0828, 1.5837) (15.1266, 1.5812) (15.1705, 1.578) (15.2144, 1.5742) (15.2583, 1.5701) (15.3023, 1.5657) (15.3463, 1.5609) (15.3903, 1.5554) (15.4343, 1.5493) (15.4783, 1.5425) (15.5224, 1.535) (15.5664, 1.527) (15.6104, 1.5186) (15.6545, 1.5097) (15.6985, 1.5005) (15.7425, 1.4909) (15.7866, 1.4808) (15.8306, 1.4704) (15.8746, 1.4595) (15.9186, 1.4482) (15.9626, 1.4365) (16.0065, 1.4244) (16.0505, 1.4119) (16.0944, 1.3991) (16.1383, 1.3859) (16.1822, 1.3724) (16.2261, 1.3585) (16.2699, 1.3443) (16.3137, 1.3297) (16.3575, 1.3147) (16.4013, 1.2995) (16.4451, 1.2839) (16.4888, 1.2679) (16.5324, 1.2517) (16.5761, 1.2351) (16.6197, 1.2182) (16.6633, 1.201) (16.7068, 1.1835) (16.7504, 1.1657) (16.7938, 1.1475) (16.8373, 1.1291) (16.8807, 1.1104) (16.924, 1.0913) (16.9674, 1.072) (17.0106, 1.0524) (17.0539, 1.0325) (17.0971, 1.0123) (17.1402, 0.9918) (17.1833, 0.9711) (17.2264, 0.95) (17.2694, 0.9287) (17.3123, 0.9071) (17.3552, 0.8852) (17.3981, 0.863) (17.4409, 0.8406) (17.4837, 0.8179) (17.5264, 0.795) (17.569, 0.7717) (17.6116, 0.7482) (17.6541, 0.7245) (17.6966, 0.7004) (17.7391, 0.6762) (17.7814, 0.6516) (17.8237, 0.6268) (17.866, 0.6018) (17.9082, 0.5765) (17.9419, 0.556) (17.9671, 0.5405) (17.9839, 0.5302) (17.9923, 0.525) knots 0 0 0 0 0 0 0.01428571 0.02857143 0.04285714 0.05714286 0.07142857 0.08571429 0.1 0.11428571 0.12857143 0.14285714 0.15714286 0.17142857 0.18571429 0.2 0.21428571 0.22857143 0.24285714 0.25714286 0.27142857 0.28571429 0.3 0.31428571 0.32857143 0.34285714 0.35714286 0.37142857 0.38571429 0.4 0.41428571 0.42857143 0.44285714 0.45714286 0.47142857 0.48571429 0.5 0.51428571 0.52857143 0.54285714 0.55714286 0.57142857 0.58571429 0.6 0.61428571 0.62857143 0.64285714 0.65714286 0.67142857 0.68571429 0.7 0.71428571 0.72857143 0.74285714 0.75714286 0.77142857 0.78571429 0.8 0.81428571 0.82857143 0.84285714 0.85714286 0.87142857 0.88571429 0.9 0.91428571 0.92857143 0.94285714 0.95714286 0.97142857 0.98571429 1 1 1 1 1 1
  arc A0 (17.9923, -0.525) -> (17.9923, 0.525) centre (0, 0) ccw
  line L0 (13.6003, -1.437) -> (14.9519, -1.5798)
  line L1 (13.6003, 1.437) -> (14.9519, 1.5798)
  line L2 (13.6003, -1.437) -> (13.6003, 1.437)
  point P0 (15.165, -1.5783)
  point P1 (15.3801, -1.5566)
  point P2 (15.5964, -1.5212)
  point P3 (15.8136, -1.4744)
  point P4 (16.0315, -1.4173)
  point P5 (16.2497, -1.3508)
  point P6 (16.4682, -1.2754)
  point P7 (16.6868, -1.1915)
  point P8 (16.9054, -1.0995)
  point P9 (17.1237, -0.9996)
  point P10 (17.3417, -0.892)
  point P11 (17.5593, -0.777)
  point P12 (17.7762, -0.6546)
  point P13 (15.165, 1.5783)
  point P14 (15.3801, 1.5566)
  point P15 (15.5964, 1.5212)
  point P16 (15.8136, 1.4744)
  point P17 (16.0315, 1.4173)
  point P18 (16.2497, 1.3508)
  point P19 (16.4682, 1.2754)
  point P20 (16.6868, 1.1915)
  point P21 (16.9054, 1.0995)
  point P22 (17.1237, 0.9996)
  point P23 (17.3417, 0.892)
  point P24 (17.5593, 0.777)
  point P25 (17.7762, 0.6546)
extrude "Extrude2'" add sketch "Gear Tooth (2)" along normal blind 10 bodies 3 in component "Sun Gear"
fillet "Fillet1'" radius 1 2 edges at (13.6102, -1.438, 5) (13.6102, 1.438, 5) on bodies 3 in component "Sun Gear"
pattern_circular "C-Pattern1'" count 16 over 360 about axis through (0, 0, 0) along (0, 0, 1) of "Extrude2'", "Fillet1'" in component "Sun Gear"
sketch "Diametrial Pitch Circle (2)" plane through (0, 0, 0) normal (0, 0, 1) x (1, 0, 0) in component "Sun Gear"
  circle A0 centre (0, 0) radius 16 construction